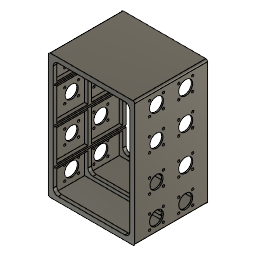
box 3d model (Autodesk Fusion 360 design; units mm, degrees)
Autodesk Fusion 360 part; units mm, degrees
note: some values were not read from the file. Set by a fixed rule: which sketch regions a step uses.
sketch "Sketch1" plane through (0, 0, 0) normal (0, 1, 0) x (1, 0, 0)
  line L0 (-62, 90) -> (62, 90)
  line L1 (62, 90) -> (62, -90)
  line L2 (62, -90) -> (-62, -90)
  line L3 (-62, -90) -> (-62, 90)
  line L4 (-62, 90) -> (62, -90) construction
  line L5 (62, 90) -> (-62, -90) construction
  line L6 (-60, 88) -> (60, 88)
  line L7 (60, 88) -> (60, -88)
  line L8 (60, -88) -> (-60, -88)
  line L9 (-60, -88) -> (-60, 88)
  line L10 (-55, 83) -> (55, 83)
  line L11 (55, 83) -> (55, -83)
  line L12 (55, -83) -> (-55, -83)
  line L13 (-55, -83) -> (-55, 83)
  line L14 (-60, 1.2) -> (60, 1.2)
  line L15 (60, 1.2) -> (60, -1.2)
  line L16 (60, -1.2) -> (-60, -1.2)
  line L17 (-60, -1.2) -> (-60, 1.2)
  line L18 (-60, 1.2) -> (60, -1.2) construction
  line L19 (60, 1.2) -> (-60, -1.2) construction
  line L20 (60, -3.2) -> (-60, -3.2)
  line L21 (-60, 3.2) -> (60, 3.2)
  line L22 (-60, 48.2) -> (60, 48.2)
  line L23 (60, 48.2) -> (60, 54.6)
  line L24 (60, 54.6) -> (-60, 54.6)
  line L25 (-60, 54.6) -> (-60, 48.2)
  line L26 (-60, 50.2) -> (60, 50.2)
  line L27 (60, 50.2) -> (60, 52.6)
  line L28 (60, 52.6) -> (-60, 52.6)
  line L29 (-60, 52.6) -> (-60, 50.2)
  line L30 (-60, -54.2) -> (60, -54.2)
  line L31 (60, -54.2) -> (60, -48.2)
  line L32 (60, -48.2) -> (-60, -48.2)
  line L33 (-60, -48.2) -> (-60, -54.2)
  line L34 (-60, -52.2) -> (60, -52.2)
  line L35 (60, -52.2) -> (60, -50.2)
  line L36 (60, -50.2) -> (-60, -50.2)
  line L37 (-60, -50.2) -> (-60, -52.2)
  dimension "d2" = 180
  dimension "d3" = 2
  dimension "d4" = 5
  dimension "d5" = 2.4
  dimension "d6" = -2
  dimension "d7" = -2
  dimension "d64" = 120
  dimension "d82" = 2
  dimension "d83" = 2
  dimension "d84" = 2.4
  dimension "d85" = 45
  dimension "d86" = 2
  dimension "d87" = 2
  dimension "d88" = 2
  dimension "d89" = 45
  constraint horizontal L0
  constraint perpendicular L0 L1
  constraint parallel L0 L2
  constraint parallel L1 L3
  constraint coincident L4 origin
  constraint coincident L5 origin
  constraint horizontal L14
  constraint perpendicular L14 L15
  constraint parallel L14 L16
  constraint parallel L15 L17
  constraint coincident L18 origin
  constraint coincident L19 origin
  constraint coincident L9 L14.start
  constraint coincident L9 L21.start
  constraint coincident L7 L20.start
  constraint horizontal L22
  constraint vertical L23
  constraint horizontal L24
  constraint vertical L25
  constraint coincident L7 L23.end
  constraint coincident L9 L22.start
  constraint horizontal L26
  constraint vertical L27
  constraint horizontal L28
  constraint vertical L29
  constraint coincident L7 L27.end
  constraint coincident L9 L26.start
  constraint horizontal L30
  constraint vertical L31
  constraint horizontal L32
  constraint vertical L33
  constraint coincident L7 L31.end
  constraint coincident L9 L30.start
  constraint horizontal L34
  constraint vertical L35
  constraint horizontal L36
  constraint vertical L37
  constraint coincident L7 L35.end
  constraint coincident L33 L34.start
  measures "d2" distance of L0.end L1.end
  measures "d5" distance of L14.end L15.end
  measures "d64" distance of L7 L9
  measures "d82" distance of L22 L26
  measures "d83" distance of L24 L28
  measures "d84" distance of L26 L28
  measures "d85" distance of L21 L22
  measures "d86" distance of L30 L34
  measures "d87" distance of L34 L36
  measures "d88" distance of L32 L36
  measures "d89" distance of L20 L32
extrude "Extrude1" add sketch "Sketch1" along normal blind 105 contours L0 L1 L2 L3 | L9 L13 L24 L25 L28 | L7 L11 L23 L24 L28 | L9 L13 L22 L25 L26 | L7 L11 L22 L23 L26 | L9 L13 L14 L21 | L7 L11 L14 L21 | L9 L13 L16 L20 | L7 L11 L16 L20 | L9 L13 L32 L33 L36 | L7 L11 L31 L32 L36 | L9 L13 L30 L33 L34 | L7 L11 L30 L31 L34 makes body 1
sketch "Sketch3" plane through (-62, 0, 0) normal (-1, 0, 0) x (0, -1, 0)
  line L0 (0, -90) -> (0, 90)
  line L1 (0, 90) -> (-105, 90)
  line L2 (-105, 90) -> (-105, -90)
  line L3 (-105, -90) -> (0, -90)
  line L4 (0, 0) -> (-105, 0)
  line L5 (-61, 38.2) -> (-86, 38.2)
  line L6 (-86, 38.2) -> (-86, 13.2)
  line L7 (-86, 13.2) -> (-61, 13.2)
  line L8 (-61, 13.2) -> (-61, 38.2)
  circle A0 centre (-83.5, 35.7) radius 1.6
  circle A1 centre (-63.5, 35.7) radius 1.6
  circle A2 centre (-83.5, 15.7) radius 1.6
  circle A3 centre (-63.5, 15.7) radius 1.6
  circle A4 centre (-73.5, 25.7) radius 10
  line L9 (-52.5, 90) -> (-52.5, -90)
  line L10 (-19, 38.2) -> (-19, 13.2)
  circle A5 centre (-21.5, 35.7) radius 1.6
  circle A6 centre (-31.5, 25.7) radius 9.3333
  line L11 (-44, 38.2) -> (-19, 38.2)
  circle A7 centre (-41.5, 35.7) radius 1.6
  line L12 (-44, 13.2) -> (-44, 38.2)
  circle A8 centre (-41.5, 15.7) radius 1.6
  line L13 (-19, 13.2) -> (-44, 13.2)
  circle A9 centre (-21.5, 15.7) radius 1.6
  line L14 (-105, 51) -> (0, 51)
  circle A10 centre (-21.5, -35.7) radius 1.6
  circle A11 centre (-31.5, -25.7) radius 9.3333
  circle A12 centre (-41.5, -35.7) radius 1.6
  line L15 (-52.5, -90) -> (-52.5, 90)
  line L16 (-44, -13.2) -> (-44, -38.2)
  line L17 (-19, -13.2) -> (-44, -13.2)
  line L18 (-61, -13.2) -> (-61, -38.2)
  circle A13 centre (-21.5, -15.7) radius 1.6
  circle A14 centre (-63.5, -15.7) radius 1.6
  line L19 (-61, -38.2) -> (-86, -38.2)
  circle A15 centre (-63.5, -35.7) radius 1.6
  circle A16 centre (-41.5, -15.7) radius 1.6
  circle A17 centre (-73.5, -25.7) radius 10
  circle A18 centre (-83.5, -35.7) radius 1.6
  circle A19 centre (-83.5, -15.7) radius 1.6
  line L20 (-86, -38.2) -> (-86, -13.2)
  line L21 (-44, -38.2) -> (-19, -38.2)
  line L22 (-86, -13.2) -> (-61, -13.2)
  line L23 (-19, -38.2) -> (-19, -13.2)
  line L24 (-19, 83.2) -> (-19, 58.2)
  circle A20 centre (-21.5, 60.7) radius 1.6
  line L25 (-86, 58.2) -> (-61, 58.2)
  circle A21 centre (-63.5, 60.7) radius 1.6
  circle A22 centre (-63.5, 80.7) radius 1.6
  line L26 (-61, 83.2) -> (-86, 83.2)
  circle A23 centre (-73.5, 70.7) radius 10
  line L27 (-19, 58.2) -> (-44, 58.2)
  circle A24 centre (-83.5, 60.7) radius 1.6
  circle A25 centre (-41.5, 80.7) radius 1.6
  line L28 (-61, 58.2) -> (-61, 83.2)
  line L29 (-52.5, 135) -> (-52.5, -45)
  circle A26 centre (-31.5, 70.7) radius 10
  line L30 (-52.5, -45) -> (-52.5, 135)
  circle A27 centre (-83.5, 80.7) radius 1.6
  line L31 (-86, 83.2) -> (-86, 58.2)
  line L32 (-44, 83.2) -> (-19, 83.2)
  line L33 (-44, 58.2) -> (-44, 83.2)
  circle A28 centre (-41.5, 60.7) radius 1.6
  circle A29 centre (-21.5, 80.7) radius 1.6
  line L34 (-61, -58.2) -> (-61, -83.2)
  line L35 (-86, -83.2) -> (-86, -58.2)
  circle A30 centre (-41.5, -80.7) radius 1.6
  line L36 (-19, -58.2) -> (-44, -58.2)
  line L37 (-52.5, -135) -> (-52.5, 45)
  circle A31 centre (-21.5, -80.7) radius 1.6
  circle A32 centre (-83.5, -60.7) radius 1.6
  line L38 (-86, -58.2) -> (-61, -58.2)
  circle A33 centre (-41.5, -60.7) radius 1.6
  line L39 (-44, -58.2) -> (-44, -83.2)
  circle A34 centre (-63.5, -80.7) radius 1.6
  line L40 (-52.5, 45) -> (-52.5, -135)
  line L41 (-61, -83.2) -> (-86, -83.2)
  line L42 (-19, -83.2) -> (-19, -58.2)
  circle A35 centre (-63.5, -60.7) radius 1.6
  circle A36 centre (-83.5, -80.7) radius 1.6
  line L43 (-52.5, 90) -> (-52.5, -90)
  circle A37 centre (-21.5, -60.7) radius 1.6
  line L44 (-52.5, -90) -> (-52.5, 90)
  circle A38 centre (-31.5, -70.7) radius 10
  circle A39 centre (-73.5, -70.7) radius 10
  line L45 (-44, -83.2) -> (-19, -83.2)
  point P0 (-73.5, 25.7)
  point P1 (-105, 48.2)
  point P2 (-105, 3.2)
  point P3 (-73.5, -25.7)
  point P4 (-73.5, 70.7)
  dimension "d10" = 180
  dimension "d11" = 105
  dimension "d19" = 25
  dimension "d20" = 25
  dimension "d21" = 19
  dimension "d31" = 3.2
  dimension "d32" = 3.2
  dimension "d33" = 3.2
  dimension "d34" = 3.2
  dimension "d35" = 20
  dimension "d90" = 25
  dimension "d92" = 52.5
  dimension "d93" = 45
  dimension "d94" = 12.5
  dimension "d95" = 2.5
  dimension "d96" = 2.5
  dimension "d97" = 2.5
  dimension "d98" = 2.5
  dimension "d99" = 25.7
  dimension "d100" = 17
  dimension "d115" = 2.5
  dimension "d116" = 2.5
  dimension "d117" = 2.5
  dimension "d118" = 2.5
  dimension "d119" = 25
  dimension "d120" = 25
  dimension "d121" = 3.2
  dimension "d122" = 3.2
  dimension "d123" = 3.2
  dimension "d124" = 3.2
  dimension "d125" = 20
  dimension "d126" = 25
  dimension "d127" = 12.5
  dimension "d128" = 2.5
  dimension "d129" = 2.5
  dimension "d130" = 2.5
  dimension "d131" = 2.5
  dimension "d132" = 17
  dimension "d133" = 2.5
  dimension "d134" = 2.5
  dimension "d135" = 2.5
  dimension "d136" = 2.5
  dimension "d137" = 12.5
  dimension "d138" = 12.5
  dimension "d139" = 12.5
  dimension "d140" = 12.5
  dimension "d142" = 12.5
  dimension "d143" = 12.5
  constraint coincident L4.start origin
  constraint midpoint L2 L4.end
  constraint horizontal L5
  constraint perpendicular L5 L6
  constraint parallel L5 L7
  constraint parallel L6 L8
  constraint coincident P0 A4.centre
  constraint coincident L1 L9.start
  constraint coincident L3 L9.end
  constraint perpendicular L3 L9
  constraint symmetric L5.end L9 L10.start
  constraint symmetric L6.end L9 L10.end
  constraint symmetric L7.end L9 L12.start
  constraint symmetric A0 L9 A5
  constraint symmetric A1 L9 A7
  constraint symmetric A2 L9 A9
  constraint symmetric A3 L9 A8
  constraint coincident L2 L14.start
  constraint coincident L0 L14.end
  constraint perpendicular L0 L14
  constraint symmetric L4 L5.start L18.end
  constraint symmetric L4 L5.end L19.end
  constraint symmetric L4 L6.end L20.end
  constraint symmetric L4 L7.end L18.start
  constraint symmetric L4 P0 P3
  constraint symmetric L4 A0 A18
  constraint symmetric L4 A1 A15
  constraint symmetric L4 A2 A19
  constraint symmetric L4 A3 A14
  constraint symmetric L4 A4 A17
  constraint symmetric L4 L9.start L9.end
  constraint symmetric L4 L9.end L9.start
  constraint symmetric L4 L10.start L21.end
  constraint symmetric L4 L10.end L17.start
  constraint symmetric L4 A5 A10
  constraint symmetric L4 A6 A11
  constraint symmetric L4 L11.start L16.end
  constraint symmetric L4 A7 A12
  constraint symmetric L4 L12.start L16.start
  constraint symmetric L4 A8 A16
  constraint symmetric L4 A9 A13
  constraint horizontal L26
  constraint perpendicular L26 L31
  constraint parallel L25 L26
  constraint parallel L28 L31
  constraint coincident P4 A23.centre
  constraint symmetric L26.end L24.start L29
  constraint symmetric L25.start L24.end L29
  constraint symmetric L25.end L27.end L29
  constraint symmetric L29 A27 A29
  constraint symmetric A22 A25 L29
  constraint symmetric A20 A24 L29
  constraint symmetric A21 L29 A28
  measures "d10" distance of L0.start L0.end
  measures "d11" distance of L0.end L1.end
  measures "d19" distance of L6.end L7.end
  measures "d20" distance of L5.end L6.end
  measures "d21" distance of L2 L6
  measures "d31" diameter of A0
  measures "d32" diameter of A1
  measures "d33" diameter of A2
  measures "d34" diameter of A3
  measures "d35" diameter of A4
  measures "d90" distance of L5.start L5.end
  measures "d92" distance of L0 L9
  measures "d93" distance of P1 P2
  measures "d94" distance of L5 P0
  measures "d95" distance of L5 A0.centre
  measures "d96" distance of L5 A1.centre
  measures "d97" distance of L7 A3.centre
  measures "d98" distance of L7 A2.centre
  measures "d99" distance of L4 P0
  measures "d100" distance of L8 L12
  measures "d115" distance of L6 A0.centre
  measures "d116" distance of L8 A1.centre
  measures "d117" distance of L8 A3.centre
  measures "d118" distance of L6 A2.centre
  measures "d119" distance of L25.end L25.start
  measures "d120" distance of L26.end L25.start
  measures "d121" diameter of A27
  measures "d122" diameter of A22
  measures "d123" diameter of A24
  measures "d124" diameter of A21
  measures "d125" diameter of A23
  measures "d126" distance of L26.end L26.start
  measures "d127" distance of P4 L26
  measures "d128" distance of A27.centre L26
  measures "d129" distance of A22.centre L26
  measures "d130" distance of A21.centre L25
  measures "d131" distance of A24.centre L25
  measures "d132" distance of L28 L33
  measures "d133" distance of A27.centre L31
  measures "d134" distance of A22.centre L28
  measures "d135" distance of A21.centre L28
  measures "d136" distance of A24.centre L31
  measures "d137" distance of L8 P0
  measures "d138" distance of P4 L28
  measures "d139" distance of A26.centre L24
  measures "d140" distance of L10 A6.centre
  measures "d142" distance of A38.centre L42
  measures "d143" distance of A39.centre L34
extrude "Extrude2" cut sketch "Sketch3" against normal blind 120 contours A0 | A1 | A2 | A3 | A4 bodies 1
fillet "Fillet3" radius 2.5 4 edges at (-62, 52.5, 90) (62, 52.5, 90) (-62, 52.5, -90) (62, 52.5, -90) on bodies 1
extrude "Extrude15" cut sketch "Sketch3" against normal blind 125 contours A0 | A1 | A2 | A3 | A4 | A5 | A6 | A7 | A8 | A9 | A10 | A11 | A12 | A13 | A14 | A15 | A16 | A17 | A18 | A19 | A20 | A21 | A22 | A23 | A24 | A25 | A26 | A27 | A28 | A29 | A30 | A31 | A32 | A33 | A34 | A35 | A36 | A37 | A38 | A39 bodies 1
extrude "Extrude17" add sketch "Sketch1" along normal blind 105 separate body contours L6 L7 L9 L10 L11 L13 L24 | L9 L13 L21 L22 | L7 L11 L21 L22 | L9 L13 L20 L32 | L7 L11 L20 L32 | L7 L8 L9 L11 L12 L13 L30 makes body 2 at (60, 70, -18.2) makes body 3 at (20, 70, 88) makes body 4 at (-55, 35, -18.2) makes body 5 at (60, 35, 18.2) makes body 6 at (-60, 35, 33.2) makes body 7 at (-20, 70, -88)
extrude "Extrude19" cut sketch "Sketch1" along normal blind 100 contours L6 L7 L9 L10 L11 L13 L24 | L9 L13 L21 L22 | L7 L11 L21 L22 | L9 L13 L20 L32 | L7 L11 L20 L32 | L7 L8 L9 L11 L12 L13 L30 bodies 2 3 4 5 6 7
extrude "Extrude20" add sketch "Sketch1" along normal blind 55 contours L6 L7 L9 L10 L11 L13 L24 | L9 L13 L21 L22 | L7 L11 L21 L22 | L9 L13 L20 L32 | L7 L11 L20 L32 | L7 L8 L9 L11 L12 L13 L30 bodies 1
extrude "Extrude21" cut sketch "Sketch1" along normal blind 50 contours L6 L7 L9 L10 L11 L13 L24 | L9 L13 L21 L22 | L7 L11 L21 L22 | L9 L13 L20 L32 | L7 L11 L20 L32 | L7 L8 L9 L11 L12 L13 L30 bodies 1
extrude "Extrude22" add sketch "Sketch1" along normal blind 5 contours L6 L7 L9 L10 L11 L13 L24 | L9 L13 L21 L22 | L7 L11 L21 L22 | L9 L13 L20 L32 | L7 L11 L20 L32 | L7 L8 L9 L11 L12 L13 L30 bodies 1
extrude "Extrude23" add sketch "Sketch1" along normal blind 2.25 contours L9 L13 L25 L26 L28 L29 | L7 L11 L23 L26 L27 L28 | L9 L13 L14 L16 L17 | L7 L11 L14 L15 L16 | L9 L13 L33 L34 L36 L37 | L7 L11 L31 L34 L35 L36 bodies 1
fillet "Fillet4" radius 7 12 edges at (-55, 52.5, -83) (-55, 2.5, -83) (55, 52.5, -83) (55, 2.5, -83) (-55, 2.5, 83) (-55, 52.5, 83) (55, 2.5, 83) (55, 52.5, 83) (-55, 102.5, 83) (55, 102.5, 83) (-55, 102.5, -83) (55, 102.5, -83) on bodies 1 3 7
combine "Combine2" operation add target body 1 tool bodies 2 6 5 3 7 4
equation "d92 = ( 105 / 2 ) * 1 mm"
equation "d99 = ( ( 45 / 2 ) * 1 mm ) + 2 mm + ( 2.4 / 2 ) * 1 mm"
equation "d148 = 105 mm - 5 mm"
equation "d150 = ( 105 / 2 ) * 1 mm + 2.5 mm"
equation "d152 = ( 105 / 2 ) * 1 mm - 2.5 mm"
equation "d156 = ( ( 100 - 95.5 ) / 2 ) * 1 mm"
